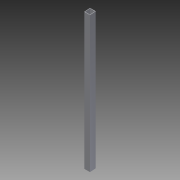
# Autodesk Inventor part: Square Tube 5
Saved by Autodesk Inventor 2013 (Build 170138000, 138)
## iProperties
Created: 2013-01-25
Part Number: Square Tube 5
Material: Aluminum 6061
Document SubType Name: Modeling
Designer: Arpan
Mass: 245.48 g
Surface Area: 1144.24 cm^2
Volume: 90.5832 cm^3
Density: 2.71 g/cm^3
Author: Arpan
Autodesk Inventor part; units mm, degrees
ref_plane "YZ Plane" through (0, 0, 0) normal (1, 0, 0) x (0, 1, 0)
ref_plane "XZ Plane" through (0, 0, 0) normal (0, 1, 0) x (-1, 0, 0)
ref_plane "XY Plane" through (0, 0, 0) normal (0, 0, 1) x (1, 0, 0)
sketch "Sketch1" plane through (0, 0, 0) normal (0, 1, 0) x (-1, 0, 0)
  line L0 (0, 0) -> (-25.4, 0)
  line L1 (-25.4, 0) -> (-25.4, 25.4)
  line L2 (-25.4, 25.4) -> (0, 25.4)
  line L3 (0, 25.4) -> (0, 0)
  line L4 (-1.5875, 1.5875) -> (-23.8125, 1.5875)
  line L5 (-23.8125, 1.5875) -> (-23.8125, 23.8125)
  line L6 (-23.8125, 23.8125) -> (-1.5875, 23.8125)
  line L7 (-1.5875, 23.8125) -> (-1.5875, 1.5875)
  dimension "d0" = 25.4
  dimension "d2" = 25.4
  dimension "d3" = 1.5875
  constraints: 16 end point, 4 parallel, 2 perpendicular, 1 horizontal, 3 other
  measures "d0" distance of L1.end L2.end
  measures "d2" distance of L2.end L0.start
  measures "d3" distance between parallel lines of L3 L7
extrude "Extrusion1" add sketch "Sketch1" along normal blind 762
sketch "Sketch2" plane through (25.4, 0, 25.4) normal (1, 0, 0) x (0, 0, -1)
  line L0 (25.4, 0) -> (0, 0) projected
  line L1 (25.4, 0) -> (25.4, 762) projected
  line L2 (0, 762) -> (25.4, 762) projected
  line L3 (0, 0) -> (0, 762) projected
  line L4 (0, 0) -> (25.4, 2.1617)
  line L5 (0, 599.0578) -> (25.4, 601.2195)
  dimension "d6" = 596.9
  dimension "d8" = 599.0578
  constraints: 4 end point, 3 point on line, 1 parallel
  measures "d6" distance between parallel lines of L4 L5
  measures "d8" distance of L0.end L5.start
extrude "Extrusion2" cut sketch "Sketch2" against normal blind 762 contours L0 L4 L1 | L3 L2 L1 L5
body "Solid1"
